Autodesk Inventor part; units mm, degrees
(part 2 of 2)
  line L567 (42.75, 0.9881) -> (40.25, -3.342)
  line L568 (40.25, -3.342) -> (35.25, -3.342)
  line L569 (35.25, -3.342) -> (32.75, 0.9881)
  line L570 (5.25, -46.6432) -> (7.75, -42.3131)
  line L571 (7.75, -42.3131) -> (12.75, -42.3131)
  line L572 (12.75, -42.3131) -> (15.25, -46.6432)
  line L573 (15.25, -46.6432) -> (12.75, -50.9734)
  line L574 (12.75, -50.9734) -> (7.75, -50.9734)
  line L575 (7.75, -50.9734) -> (5.25, -46.6432)
  line L576 (38.25, 10.5144) -> (40.75, 14.8446)
  line L577 (40.75, 14.8446) -> (45.75, 14.8446)
  line L578 (45.75, 14.8446) -> (48.25, 10.5144)
  line L579 (48.25, 10.5144) -> (45.75, 6.1843)
  line L580 (45.75, 6.1843) -> (40.75, 6.1843)
  line L581 (40.75, 6.1843) -> (38.25, 10.5144)
  line L582 (-0.25, -56.1695) -> (2.25, -51.8394)
  line L583 (2.25, -51.8394) -> (7.25, -51.8394)
  line L584 (7.25, -51.8394) -> (9.75, -56.1695)
  line L585 (9.75, -56.1695) -> (7.25, -60.4997)
  line L586 (7.25, -60.4997) -> (2.25, -60.4997)
  line L587 (2.25, -60.4997) -> (-0.25, -56.1695)
  line L588 (43.75, 20.0407) -> (46.25, 24.3708)
  line L589 (46.25, 24.3708) -> (51.25, 24.3708)
  line L590 (51.25, 24.3708) -> (53.75, 20.0407)
  line L591 (53.75, 20.0407) -> (51.25, 15.7106)
  line L592 (51.25, 15.7106) -> (46.25, 15.7106)
  line L593 (46.25, 15.7106) -> (43.75, 20.0407)
  line L594 (-5.75, -65.6958) -> (-3.25, -61.3657)
  line L595 (-3.25, -61.3657) -> (1.75, -61.3657)
  line L596 (1.75, -61.3657) -> (4.25, -65.6958)
  line L597 (4.25, -65.6958) -> (1.75, -70.0259)
  line L598 (1.75, -70.0259) -> (-3.25, -70.0259)
  line L599 (-3.25, -70.0259) -> (-5.75, -65.6958)
  point P0 (15, 0)
  point P1 (-0.75, 29.567)
  point P2 (-6.25, 20.0407)
  point P3 (4.75, 39.0933)
  point P4 (-11.75, 10.5144)
  point P5 (10.25, 48.6195)
  point P6 (-17.25, 0.9881)
  point P7 (15.75, 58.1458)
  point P8 (-22.75, -8.5381)
  point P9 (21.25, 67.6721)
  point P10 (-28.25, -18.0644)
  point P11 (4.75, 20.0407)
  point P12 (-0.75, 10.5144)
  point P13 (10.25, 29.567)
  point P14 (-6.25, 0.9881)
  point P15 (15.75, 39.0933)
  point P16 (-11.75, -8.5381)
  point P17 (21.25, 48.6195)
  point P18 (-17.25, -18.0644)
  point P19 (26.75, 58.1458)
  point P20 (-22.75, -27.5907)
  point P21 (-6.25, 39.0933)
  point P22 (-11.75, 29.567)
  point P23 (-0.75, 48.6195)
  point P24 (-17.25, 20.0407)
  point P25 (4.75, 58.1458)
  point P26 (-22.75, 10.5144)
  point P27 (10.25, 67.6721)
  point P28 (-28.25, 0.9881)
  point P29 (15.75, 77.1984)
  point P30 (-33.75, -8.5381)
  point P31 (10.25, 10.5144)
  point P32 (4.75, 0.9881)
  point P33 (15.75, 20.0407)
  point P34 (-0.75, -8.5381)
  point P35 (21.25, 29.567)
  point P36 (-6.25, -18.0644)
  point P37 (26.75, 39.0933)
  point P38 (-11.75, -27.5907)
  point P39 (32.25, 48.6195)
  point P40 (-17.25, -37.117)
  point P41 (-11.75, 48.6195)
  point P42 (-17.25, 39.0933)
  point P43 (-6.25, 58.1458)
  point P44 (-22.75, 29.567)
  point P45 (-0.75, 67.6721)
  point P46 (-28.25, 20.0407)
  point P47 (4.75, 77.1984)
  point P48 (-33.75, 10.5144)
  point P49 (10.25, 86.7247)
  point P50 (-39.25, 0.9881)
  point P51 (15.75, 0.9881)
  point P52 (10.25, -8.5381)
  point P53 (21.25, 10.5144)
  point P54 (4.75, -18.0644)
  point P55 (26.75, 20.0407)
  point P56 (-0.75, -27.5907)
  point P57 (32.25, 29.567)
  point P58 (-6.25, -37.117)
  point P59 (37.75, 39.0933)
  point P60 (-11.75, -46.6432)
  point P61 (-17.25, 58.1458)
  point P62 (-22.75, 48.6195)
  point P63 (-11.75, 67.6721)
  point P64 (-28.25, 39.0933)
  point P65 (-6.25, 77.1984)
  point P66 (-33.75, 29.567)
  point P67 (-0.75, 86.7247)
  point P68 (-39.25, 20.0407)
  point P69 (4.75, 96.2509)
  point P70 (-44.75, 10.5144)
  point P71 (21.25, -8.5381)
  point P72 (15.75, -18.0644)
  point P73 (26.75, 0.9881)
  point P74 (10.25, -27.5907)
  point P75 (32.25, 10.5144)
  point P76 (4.75, -37.117)
  point P77 (37.75, 20.0407)
  point P78 (-0.75, -46.6432)
  point P79 (43.25, 29.567)
  point P80 (-6.25, -56.1695)
  point P81 (-22.75, 67.6721)
  point P82 (-28.25, 58.1458)
  point P83 (-17.25, 77.1984)
  point P84 (-33.75, 48.6195)
  point P85 (-11.75, 86.7247)
  point P86 (-39.25, 39.0933)
  point P87 (-6.25, 96.2509)
  point P88 (-44.75, 29.567)
  point P89 (-0.75, 105.7772)
  point P90 (-50.25, 20.0407)
  point P91 (26.75, -18.0644)
  point P92 (21.25, -27.5907)
  point P93 (32.25, -8.5381)
  point P94 (15.75, -37.117)
  point P95 (37.75, 0.9881)
  point P96 (10.25, -46.6432)
  point P97 (43.25, 10.5144)
  point P98 (4.75, -56.1695)
  point P99 (48.75, 20.0407)
  point P100 (-0.75, -65.6958)
  dimension "d209" = 5
  dimension "d212" = 11
  dimension "d215" = 11
  constraints: 1200 end point, 2 collinear, 1300 other
  measures "d209" distance of L1.end L2.end
  measures "d212" distance of point (-0.75, 29.567) point (-6.25, 20.041)
  measures "d215" distance of point (-0.75, 29.567) point (4.75, 20.041)
extrude "Wyciągnięcie proste28" [suppressed]
